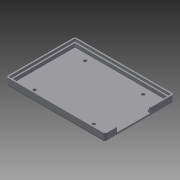
# Autodesk Inventor part: hubtest1_4
Saved by Autodesk Inventor 2015 (Build 190159000, 159)
## iProperties
Created: 2015-11-05
Part Number: hubtest1_4
Material: Generic
Document SubType Name: Modeling
Designer: mca20
Density: 1 g/cm^3
Appearance: Default
Author: mca20
Autodesk Inventor part; units mm, degrees
ref_plane "YZ Plane" through (0, 0, 0) normal (1, 0, 0) x (0, 1, 0)
ref_plane "XZ Plane" through (0, 0, 0) normal (0, 1, 0) x (-1, 0, 0)
ref_plane "XY Plane" through (0, 0, 0) normal (0, 0, 1) x (1, 0, 0)
sketch "Sketch1" plane through (0, 0, 0) normal (0, 1, 0) x (-1, 0, 0)
  line L0 (0, 0) -> (-92, 0)
  line L1 (-92, 0) -> (-92, -64)
  line L2 (-92, -64) -> (0, -64)
  line L3 (0, -64) -> (0, 0)
  dimension "d0" = 64
  dimension "d1" = 92
  constraints: 8 end point, 2 parallel, 1 horizontal, 1 perpendicular
  measures "d0" distance between parallel lines of L2 L0
  measures "d1" distance between parallel lines of L1 L3
extrude "Extrusion1" add sketch "Sketch1" along normal blind 7.5
sketch "Sketch2" plane through (0, 7.5, 0) normal (0, 1, 0) x (1, 0, 0)
  line L0 (2.5, 2.5) -> (89.5, 2.5)
  line L1 (89.5, 2.5) -> (89.5, 61.5)
  line L2 (89.5, 61.5) -> (2.5, 61.5)
  line L3 (2.5, 61.5) -> (2.5, 2.5)
  line L4 (0, 64) -> (0, 0) projected
  line L5 (0, 0) -> (92, 0) projected
  line L6 (92, 0) -> (92, 64) projected
  line L7 (92, 64) -> (0, 64) projected
  dimension "d4" = 2.5
  dimension "d5" = 2.5
  dimension "d6" = 2.5
  dimension "d7" = 2.5
  constraints: 8 end point, 2 parallel, 1 horizontal, 1 perpendicular
  measures "d4" distance between parallel lines of L4 L3
  measures "d5" distance between parallel lines of L5 L0
  measures "d6" distance between parallel lines of L6 L1
  measures "d7" distance between parallel lines of L7 L2
extrude "Extrusion2" cut sketch "Sketch2" against normal blind 6 contours L3 L2 L1 L0
fillet "Fillet1" radius 2 8 edges at (0, 3.75, 0) (46, 0, 0) (92, 3.75, 0) (92, 0, -32) (92, 3.75, -64) (46, 0, -64) (0, 3.75, -64) (0, 0, -32)
sketch "Sketch3" plane through (0, 7.5, 0) normal (0, 1, 0) x (1, 0, 0)
  line L0 (1.25, 1.25) -> (90.75, 1.25)
  line L1 (90.75, 1.25) -> (90.75, 62.75)
  line L2 (90.75, 62.75) -> (1.25, 62.75)
  line L3 (1.25, 62.75) -> (1.25, 1.25)
  line L4 (0, 62) -> (0, 2) projected
  line L5 (2, 0) -> (90, 0) projected
  line L6 (92, 2) -> (92, 62) projected
  line L7 (90, 64) -> (2, 64) projected
  point P0 (0, 0)
  dimension "d11" = 1.25
  dimension "d12" = 1.25
  dimension "d13" = 1.25
  dimension "d14" = 1.25
  constraints: 8 end point, 2 parallel, 1 horizontal, 1 perpendicular
  measures "d11" distance between parallel lines of L3 L4
  measures "d12" distance between parallel lines of L5 L0
  measures "d13" distance between parallel lines of L6 L1
  measures "d14" distance between parallel lines of L7 L2
extrude "Extrusion3" cut sketch "Sketch3" against normal blind 2.5
sketch "Sketch4" plane through (0, 1.5, 0) normal (0, 1, 0) x (1, 0, 0)
  line L0 (5, 5) -> (87, 5)
  line L1 (87, 5) -> (87, 59) construction
  line L2 (87, 59) -> (5, 59)
  line L3 (5, 59) -> (5, 5)
  line L4 (2.5, 2.5) -> (2.5, 61.5) projected
  line L5 (89.5, 2.5) -> (2.5, 2.5) projected
  line L6 (2.5, 61.5) -> (89.5, 61.5) projected
  line L7 (89.5, 61.5) -> (89.5, 2.5) projected
  line L8 (18, 55.5) -> (73, 55.5)
  line L9 (73, 55.5) -> (73, 8.5)
  line L10 (73, 8.5) -> (18, 8.5)
  line L11 (18, 8.5) -> (18, 55.5)
  line L12 (72, 55.5) -> (72, 8.5)
  point P0 (0, 0)
  dimension "d17" = 2.5
  dimension "d18" = 2.5
  dimension "d19" = 2.5
  dimension "d20" = 2.5
  dimension "d21" = 14
  dimension "d22" = 13
  dimension "d23" = 54
  dimension "d24" = 82
  dimension "d25" = 3.5
  dimension "d26" = 3.5
  dimension "d44" = 15
  dimension "d45" = 17.5
  dimension "d46" = 16.5
  constraints: 18 end point, 4 parallel, 3 perpendicular, 2 horizontal, 2 point on line
  measures "d17" distance between parallel lines of L4 L3
  measures "d18" distance between parallel lines of L5 L0
  measures "d19" distance between parallel lines of L2 L6
  measures "d20" distance between parallel lines of L7 L1
  measures "d21" distance between parallel lines of L9 L1
  measures "d22" distance between parallel lines of L11 L3
  measures "d23" distance between parallel lines of L0 L2
  measures "d24" distance between parallel lines of L1 L3
  measures "d25" distance between parallel lines of L0 L10
  measures "d26" distance between parallel lines of L2 L8
  measures "d44" distance between parallel lines of L12 L1
  measures "d45" distance between parallel lines of L7 L12
  measures "d46" distance between parallel lines of L7 L9
hole "Hole1" at (18, 1.5, -55.5) at (18, 1.5, -8.5) at (73, 1.5, -8.5) at (72, 1.5, -55.5) direction (0, -1, 0) diameter 3 end through all
sketch "Sketch5" plane through (92, 2, -2) normal (1, 0, 0) x (0, 0, -1)
  line L0 (9, 5.5) -> (40, 5.5)
  line L1 (40, 5.5) -> (40, 1)
  line L2 (40, 1) -> (9, 1)
  line L3 (9, 1) -> (9, 5.5)
  line L4 (0, 5.5) -> (60, 5.5) projected
  line L5 (0, 0) -> (0, 5.5) projected
  line L6 (60, 5.5) -> (60, 0) projected
  line L7 (60, 0) -> (0, 0) projected
  line L8 (59.5, -0.5) -> (0.5, -0.5) projected
  point P0 (-2, -2)
  dimension "d34" = 0
  dimension "d35" = 9
  dimension "d36" = 20
  dimension "d37" = 4.5
  dimension "d41" = 5.5
  dimension "d42" = 1
  dimension "d43" = 1.5
  constraints: 8 end point, 2 parallel, 1 horizontal, 1 perpendicular
  measures "d34" distance between parallel lines of L4 L0
  measures "d35" distance between parallel lines of L5 L3
  measures "d36" distance between parallel lines of L6 L1
  measures "d37" distance between parallel lines of L2 L0
  measures "d41" distance between parallel lines of L7 L4
  measures "d42" distance between parallel lines of L7 L2
  measures "d43" distance between parallel lines of L8 L2
extrude "Extrusion4" cut sketch "Sketch5" against normal blind 2.5 contours L0 L1 L2 L3
body "Solid1"
